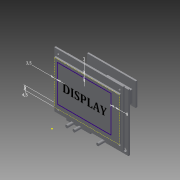
# Autodesk Inventor part: Mockup_Platinen
Saved by Autodesk Inventor 2014 (Build 180170000, 170)
## iProperties
Created: 2013-08-22
Part Number: Mockup_Platinen
Material: Generic
Document SubType Name: Modeling
Designer: md
Density: 1 g/cm^3
Appearance: Default
Author: md
Autodesk Inventor part; units mm, degrees
ref_plane "YZ Plane" through (0, 0, 0) normal (1, 0, 0) x (0, 1, 0)
ref_plane "XZ Plane" through (0, 0, 0) normal (0, 1, 0) x (-1, 0, 0)
ref_plane "XY Plane" through (0, 0, 0) normal (0, 0, 1) x (1, 0, 0)
sketch "Umriss_Sensorplatine" plane through (0, 0, 0) normal (0, 0, 1) x (1, 0, 0)
  line L0 (0, 62) -> (67, 62)
  line L1 (67, 62) -> (67, 0)
  line L2 (67, 0) -> (42, 0)
  line L3 (42, 0) -> (42, 14)
  line L4 (42, 14) -> (26, 14)
  line L5 (26, 14) -> (26, 0)
  line L6 (26, 0) -> (0, 0)
  line L7 (9, 14.3) -> (9, 25)
  line L8 (9, 25) -> (0, 25)
  line L9 (0, 0) -> (0, 9)
  line L10 (0, 25) -> (0, 62)
  circle A0 centre (63, 4) radius 2
  circle A1 centre (4, 4) radius 2
  circle A2 centre (55, 31) radius 2
  circle A3 centre (4, 58) radius 2
  line L11 (4, 4) -> (63, 4) construction
  line L12 (4, 4) -> (4, 58) construction
  line L13 (0, 9) -> (9, 14.3)
  dimension "d0" = 4
  dimension "d2" = 4
  dimension "d3" = 4
  dimension "d4" = 4
  dimension "d5" = 67
  dimension "d6" = 26
  dimension "d7" = 42
  dimension "d8" = 14
  dimension "d9" = 4
  dimension "d11" = 25
  dimension "d12" = 9
  dimension "d13" = 62
  dimension "d14" = 31
  dimension "d15" = 55
  dimension "d67" = 14.3
  dimension "d68" = 9
  constraints: 29 end point, 9 parallel, 6 perpendicular, 4 centre point, 3 equal radius, 2 collinear, 2 vertical
  measures "d0" diameter of A1
  measures "d2" distance from line of L11.start L6
  measures "d3" distance from line of L11.start L9
  measures "d4" distance from line of L11.end L1
  measures "d5" distance between parallel lines of L9 L1
  measures "d6" distance between parallel lines of L9 L5
  measures "d7" distance between parallel lines of L9 L3
  measures "d8" distance between parallel lines of L6 L4
  measures "d9" distance from line of L0 L12.end
  measures "d11" distance between parallel lines of L6 L8
  measures "d12" distance between parallel lines of L9 L7
  measures "d13" distance between parallel lines of L0 L6
  measures "d14" distance from line of L6 A2.centre
  measures "d15" distance from line of L9 A2.centre
  measures "d67" distance from line of L6 L7.start
  measures "d68" distance from line of L6 L9.end
extrude "Sensorplatine" add sketch "Umriss_Sensorplatine" along normal blind 1.75
sketch "Tasterprojektion" plane through (0, 0, 1.75) normal (0, 0, 1) x (1, 0, 0)
  line L0 (0, 0) -> (26, 0) construction
  line L1 (26, 0) -> (26, 14) construction
  line L2 (26, 14) -> (42, 14) construction
  line L3 (42, 14) -> (42, 0) construction
  line L4 (42, 0) -> (67, 0) construction
  line L5 (67, 0) -> (67, 62) construction
  line L6 (67, 62) -> (0, 62) construction
  line L7 (0, 62) -> (0, 25) construction
  line L8 (0, 9) -> (0, 0) construction
  line L9 (0, 7.3) -> (67, 7.3) construction
  circle A0 centre (13.3, 7.3) radius 1.525
  circle A1 centre (21.25, 7.3) radius 1.525
  circle A2 centre (46.75, 7.3) radius 1.525
  line L10 (43.75, 10.3) -> (49.75, 10.3)
  line L11 (49.75, 10.3) -> (49.75, 4.3)
  line L12 (49.75, 4.3) -> (43.75, 4.3)
  line L13 (43.75, 4.3) -> (43.75, 10.3)
  line L14 (43.75, 10.3) -> (49.75, 4.3) construction
  line L15 (49.75, 10.3) -> (43.75, 4.3) construction
  line L16 (18.25, 10.3) -> (24.25, 10.3)
  line L17 (24.25, 10.3) -> (24.25, 4.3)
  line L18 (24.25, 4.3) -> (18.25, 4.3)
  line L19 (18.25, 4.3) -> (18.25, 10.3)
  line L20 (18.25, 10.3) -> (24.25, 4.3) construction
  line L21 (24.25, 10.3) -> (18.25, 4.3) construction
  line L22 (10.3, 10.3) -> (16.3, 10.3)
  line L23 (16.3, 10.3) -> (16.3, 4.3)
  line L24 (16.3, 4.3) -> (10.3, 4.3)
  line L25 (10.3, 4.3) -> (10.3, 10.3)
  line L26 (10.3, 10.3) -> (16.3, 4.3) construction
  line L27 (16.3, 10.3) -> (10.3, 4.3) construction
  dimension "d19" = 7.3
  dimension "d20" = 3.05
  dimension "d21" = 13.3
  dimension "d22" = 21.25
  dimension "d23" = 46.75
  dimension "d24" = 6
  dimension "d25" = 6
  constraints: 38 end point, 6 midpoint, 6 parallel, 5 point on line, 4 equal length, 4 perpendicular, 3 centre point, 3 horizontal, 2 equal radius
  measures "d19" distance between parallel lines of L9 L0
  measures "d20" diameter of A0
  measures "d21" distance from line of L8 A0.centre
  measures "d22" distance from line of L8 A1.centre
  measures "d23" distance from line of L8 A2.centre
  measures "d24" distance of L11.end L12.end
  measures "d25" distance of L10.end L11.end
extrude "Grundkoerper Taster" add sketch "Tasterprojektion" along normal blind 3.5
extrude "Nubsis Taster" add sketch "Tasterprojektion" along normal blind 13 contours A0 | A1 | A2
sketch "Sketch3" plane through (0, 0, 1.75) normal (0, 0, 1) x (1, 0, 0)
  line L0 (37.3343, 37.5267) -> (44.9961, 37.5267)
  line L1 (44.9961, 37.5267) -> (44.9961, 54.2692)
  line L2 (44.9961, 54.2692) -> (37.3343, 54.2692)
  line L3 (37.3343, 54.2692) -> (37.3343, 37.5267)
  line L4 (37.3343, 37.5267) -> (44.9961, 54.2692) construction
  line L5 (44.9961, 37.5267) -> (37.3343, 54.2692) construction
  point P0 (41.1652, 45.898)
  constraints: 12 end point, 2 midpoint, 2 parallel, 1 horizontal, 1 perpendicular
extrude "Steckverbinder" add sketch "Sketch3" along normal blind 12
sketch "Sketch4" plane through (0, 0, 13.75) normal (0, 0, 1) x (1, 0, 0)
  line L0 (0, 62) -> (0, 25) construction
  line L1 (0, 25) -> (9, 25) construction
  line L2 (37.3343, 37.5267) -> (37.3343, 54.2692) construction
  line L3 (37.3343, 54.2692) -> (44.9961, 54.2692) construction
  line L4 (44.9961, 54.2692) -> (44.9961, 37.5267) construction
  line L5 (44.9961, 37.5267) -> (37.3343, 37.5267) construction
  line L6 (0, 0) -> (26, 0) construction
  line L7 (26, 0) -> (26, 14) construction
  line L8 (26, 14) -> (42, 14) construction
  line L9 (42, 14) -> (42, 0) construction
  line L10 (42, 0) -> (67, 0) construction
  line L11 (67, 0) -> (67, 62) construction
  line L12 (67, 62) -> (0, 62) construction
  line L13 (0, 62) -> (0, 25) construction
  line L14 (0, 25) -> (9, 25) construction
  line L15 (9, 25) -> (9, 14.3) construction
  line L16 (0, 9) -> (0, 0) construction
  circle A0 centre (63, 4) radius 2 construction
  circle A1 centre (4, 4) radius 2 construction
  circle A2 centre (55, 31) radius 2 construction
  circle A3 centre (4, 58) radius 2 construction
  line L17 (24.25, 10.3) -> (24.25, 4.3) construction
  line L18 (24.25, 4.3) -> (18.25, 4.3) construction
  line L19 (18.25, 4.3) -> (18.25, 10.3) construction
  line L20 (18.25, 10.3) -> (24.25, 10.3) construction
  line L21 (49.75, 10.3) -> (49.75, 4.3) construction
  line L22 (49.75, 4.3) -> (43.75, 4.3) construction
  line L23 (43.75, 4.3) -> (43.75, 10.3) construction
  line L24 (43.75, 10.3) -> (49.75, 10.3) construction
  line L25 (16.3, 10.3) -> (16.3, 4.3) construction
  line L26 (16.3, 4.3) -> (10.3, 4.3) construction
  line L27 (10.3, 4.3) -> (10.3, 10.3) construction
  line L28 (10.3, 10.3) -> (16.3, 10.3) construction
  line L29 (0.5, 15.5) -> (74.8, 15.5)
  line L30 (74.8, 15.5) -> (74.8, 75.5)
  line L31 (74.8, 75.5) -> (0.5, 75.5)
  line L32 (0.5, 75.5) -> (0.5, 15.5)
  line L33 (4.5, 19.5) -> (70.8, 19.5) construction
  line L34 (70.8, 19.5) -> (70.8, 71.5) construction
  line L35 (70.8, 71.5) -> (4.5, 71.5) construction
  line L36 (4.5, 71.5) -> (4.5, 19.5) construction
  circle A4 centre (70.8, 71.5) radius 1.25
  circle A5 centre (4.5, 71.5) radius 1.25
  circle A6 centre (4.5, 19.5) radius 1.25
  circle A7 centre (70.8, 19.5) radius 1.25
  line L37 (9, 14.3) -> (0, 9) projected
  dimension "d32" = 0.5
  dimension "d33" = 74.3
  dimension "d34" = 60
  dimension "d35" = 4
  dimension "d36" = 4
  dimension "d37" = 4
  dimension "d38" = 4
  dimension "d39" = 2.5
  dimension "d70" = 13.5
  dimension "d71" = 66.3
  dimension "d72" = 52
  dimension "d73" = 62
  constraints: 16 end point, 5 parallel, 4 centre point, 4 coincident, 3 equal radius, 2 perpendicular, 1 horizontal
  measures "d32" distance between parallel lines of L0 L32
  measures "d33" distance between parallel lines of L32 L30
  measures "d34" distance between parallel lines of L29 L31
  measures "d35" distance between parallel lines of L33 L29
  measures "d36" distance between parallel lines of L30 L34
  measures "d37" distance between parallel lines of L31 L35
  measures "d38" distance between parallel lines of L32 L36
  measures "d39" diameter of A4
  measures "d70" distance between parallel lines of L31 L12
  measures "d71" distance of L34.end L35.end
  measures "d72" distance of A5.centre L33.start
  measures "d73" distance between parallel lines of L6 L12
extrude "Grundplatine Display" add sketch "Sketch4" along normal blind 1.7
sketch "Sketch5" plane through (0, 0, 15.45) normal (0, 0, 1) x (1, 0, 0)
  line L0 (0.5, 15.5) -> (74.8, 15.5) projected
  line L1 (74.8, 15.5) -> (74.8, 75.5) projected
  line L2 (0.5, 75.5) -> (0.5, 15.5) projected
  circle A0 centre (70.8, 19.5) radius 1.25 construction
  circle A1 centre (4.5, 19.5) radius 1.25 construction
  circle A2 centre (4.5, 71.5) radius 1.25 construction
  circle A3 centre (70.8, 71.5) radius 1.25 construction
  line L3 (0.5, 15.5) -> (74.8, 15.5) construction
  line L4 (74.8, 15.5) -> (74.8, 75.5) construction
  line L5 (74.8, 75.5) -> (0.5, 75.5) construction
  line L6 (0.5, 75.5) -> (0.5, 15.5) construction
  line L7 (2.3, 21.5) -> (72.65, 21.5)
  line L8 (72.65, 21.5) -> (72.65, 68)
  line L9 (72.65, 68) -> (2.3, 68)
  line L10 (2.3, 68) -> (2.3, 21.5)
  point P0 (0, 0)
  dimension "d42" = 6
  dimension "d43" = 7.5
  dimension "d44" = 2.15
  dimension "d45" = 1.8
  constraints: 8 end point, 2 parallel, 1 horizontal, 1 perpendicular
  measures "d42" distance between parallel lines of L0 L7
  measures "d43" distance between parallel lines of L5 L9
  measures "d44" distance between parallel lines of L1 L8
  measures "d45" distance between parallel lines of L2 L10
extrude "Glaskoerper Display" add sketch "Sketch5" along normal blind 2
sketch "Display" plane through (0, 0, 17.45) normal (0, 0, 1) x (1, 0, 0)
  line L0 (2.3, 21.5) -> (72.65, 21.5) construction
  line L1 (72.65, 21.5) -> (72.65, 68) construction
  line L2 (72.65, 68) -> (2.3, 68) construction
  line L3 (2.3, 68) -> (2.3, 21.5) construction
  line L4 (5.8, 26) -> (63.65, 26)
  line L5 (63.65, 26) -> (63.65, 65)
  line L6 (63.65, 65) -> (5.8, 65)
  line L7 (5.8, 65) -> (5.8, 26)
  line L8 (11.3777, 48.5369) -> (83.2025, 48.5369) construction
  line L9 (83.2025, 48.5369) -> (83.2025, 36.2483) construction
  line L10 (83.2025, 36.2483) -> (11.3777, 36.2483) construction
  line L11 (11.3777, 36.2483) -> (11.3777, 48.5369) construction
  point P0 (0, 0)
  dimension "d48" = 4.5
  dimension "d49" = 3
  dimension "d50" = 9
  dimension "d51" = 3.5
  constraints: 8 end point, 2 parallel, 1 horizontal, 1 perpendicular, 2 other
  measures "d48" distance between parallel lines of L0 L4
  measures "d49" distance between parallel lines of L2 L6
  measures "d50" distance between parallel lines of L1 L5
  measures "d51" distance between parallel lines of L3 L7
extrude "Bildausschnitt" cut sketch "Display" against normal blind 0.2
sketch "Sketch7" plane through (0, 0, 0) normal (0, 0, -1) x (-1, 0, 0)
  line L0 (-66, 59.4637) -> (-39.1956, 59.4637)
  line L1 (-39.1956, 59.4637) -> (-39.1956, 46.4689)
  line L2 (-39.1956, 46.4689) -> (-66, 46.4689)
  line L3 (-66, 46.4689) -> (-66, 59.4637)
  constraints: 8 end point, 2 parallel, 1 horizontal, 1 perpendicular
extrude "Platzhalter_Stiftleiste" add sketch "Sketch7" along normal blind 3.5
sketch "Sketch8" plane through (0, 0, -3.5) normal (0, 0, -1) x (-1, 0, 0)
  line L0 (-39.1956, 59.4637) -> (-39.1956, 46.4689) construction
  line L1 (-39.1956, 46.4689) -> (-66, 46.4689) construction
  line L2 (-66, 46.4689) -> (-66, 59.4637) construction
  line L3 (-66, 59.4637) -> (-39.1956, 59.4637) construction
  circle A0 centre (-4, 58) radius 2 construction
  circle A1 centre (-55, 31) radius 2 construction
  circle A2 centre (-4, 4) radius 2 construction
  circle A3 centre (-63, 4) radius 2 construction
  line L4 (0, 0) -> (-26, 0) construction
  line L5 (0, 9) -> (0, 0) construction
  line L6 (-9, 25) -> (-9, 14.3) construction
  line L7 (0, 25) -> (-9, 25) construction
  line L8 (0, 62) -> (0, 25) construction
  line L9 (-67, 62) -> (0, 62) construction
  line L10 (-67, 0) -> (-67, 62) construction
  line L11 (-42, 0) -> (-67, 0) construction
  line L12 (-42, 14) -> (-42, 0) construction
  line L13 (-26, 14) -> (-42, 14) construction
  line L14 (-26, 0) -> (-26, 14) construction
  line L15 (-69.5, 68.6) -> (-17.1, 68.6)
  line L16 (-17.1, 68.6) -> (-17.1, 43.6)
  line L17 (-17.1, 43.6) -> (-69.5, 43.6)
  line L18 (-69.5, 43.6) -> (-69.5, 68.6)
  line L19 (-9, 14.3) -> (0, 9) projected
  dimension "d56" = 6.6
  dimension "d57" = 2.5
  dimension "d58" = 25
  dimension "d59" = 52.4
  constraints: 8 end point, 2 parallel, 1 horizontal, 1 perpendicular
  measures "d56" distance between parallel lines of L15 L9
  measures "d57" distance between parallel lines of L10 L18
  measures "d58" distance between parallel lines of L15 L17
  measures "d59" distance between parallel lines of L18 L16
extrude "HexaHorst" add sketch "Sketch8" along normal blind 1.7
sketch "Sketch9" plane through (0, 0, 0) normal (0, 0, -1) x (-1, 0, 0)
  line L0 (-67, 62) -> (0, 62) projected
  line L1 (-26, 14) -> (-42, 14) projected
  line L2 (-34, 14) -> (-33.5, 62) construction
  line L3 (-41.8906, 35) -> (-25.8906, 35)
  line L4 (-25.8906, 35) -> (-25.8906, 14)
  line L5 (-25.8906, 14) -> (-41.8906, 14)
  line L6 (-41.8906, 14) -> (-41.8906, 35)
  line L7 (-41.8906, 35) -> (-25.8906, 14) construction
  line L8 (-25.8906, 35) -> (-41.8906, 14) construction
  point P0 (-33.8906, 24.5)
  dimension "d62" = 16
  dimension "d63" = 21
  constraints: 14 end point, 4 midpoint, 2 parallel, 1 collinear, 1 horizontal, 1 perpendicular, 1 point on line
  measures "d62" distance of L4.end L5.end
  measures "d63" distance of L3.end L4.end
extrude "Extrusion10" add sketch "Sketch9" along normal blind 13.5
body "Solid1"
